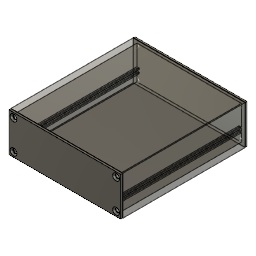
2230 Extruded aluminum box 94mm (Autodesk Fusion 360 design; units mm, degrees)
Autodesk Fusion 360 part; units mm, degrees
sketch "Sketch1" plane through (0, 0, 0) normal (0, 0, 1) x (1, 0, 0)
  line L0 (0, 0) -> (82.8, 0)
  line L1 (82.8, 0) -> (82.8, 28.8)
  line L2 (82.8, 28.8) -> (0, 28.8)
  line L3 (0, 28.8) -> (0, 0)
  line L4 (2.8, 2) -> (80, 2)
  line L5 (80, 26.8) -> (2.8, 26.8)
  line L6 (41.4, 28.8) -> (41.4, 0) construction
  line L7 (2.8, 9) -> (4.5, 9)
  line L8 (4.5, 9) -> (4.5, 8.1)
  line L9 (4.5, 8.1) -> (2.8, 8.1)
  line L10 (2.8, 8.1) -> (2.8, 9) construction
  line L11 (2.8, 11.7) -> (4.5, 11.7)
  line L12 (4.5, 11.7) -> (4.5, 10.8)
  line L13 (4.5, 10.8) -> (2.8, 10.8)
  line L14 (78.3, 8.1) -> (80, 8.1)
  line L15 (78.3, 9) -> (78.3, 8.1)
  line L16 (80, 9) -> (78.3, 9)
  line L17 (78.3, 10.8) -> (80, 10.8)
  line L18 (78.3, 11.7) -> (78.3, 10.8)
  line L19 (80, 11.7) -> (78.3, 11.7)
  line L20 (2.8, 26.8) -> (2.8, 11.7)
  line L21 (2.8, 8.1) -> (2.8, 2)
  line L22 (2.8, 10.8) -> (2.8, 9)
  line L23 (80, 11.7) -> (80, 26.8)
  line L24 (80, 2) -> (80, 8.1)
  line L25 (80, 9) -> (80, 10.8)
  dimension "d1" = 82.8
  dimension "d2" = 28.8
  dimension "d4" = 77.2
  dimension "d5" = 24.8
  dimension "d6" = 2
  dimension "d7" = 2.8
  dimension "d8" = 41.4
  dimension "d9" = 1.7
  dimension "d10" = 0.9
  dimension "d15" = 1.8
  dimension "d17" = 0.9
  dimension "d20" = 7
  measures "d4" distance of L0.start
  measures "d6" distance of L2 L5
  measures "d7" distance of L1 L24
  measures "d8" distance of L1 L6
  measures "d15" distance of L7 L13
  measures "d17" distance of L11 L13
  measures "d20" distance of L4 L7
extrude "Extrude1" add sketch "Sketch1" along normal blind 90.5 makes body 1
sketch "Sketch1 (2)" plane through (0, 0, 0) normal (0, 0, 1) x (1, 0, 0) in component "BackPanel"
  line L0 (0, 0) -> (82.8, 0)
  line L1 (82.8, 0) -> (82.8, 28.8)
  line L2 (82.8, 28.8) -> (0, 28.8)
  line L3 (0, 28.8) -> (0, 0)
  circle A0 centre (3.5, 3.5) radius 1.5
  circle A1 centre (79.3, 3.5) radius 1.5
  circle A2 centre (3.5, 25.3) radius 1.5
  circle A3 centre (79.3, 25.3) radius 1.5
  line L4 (0, 0) -> (3.5, 3.5) construction
  line L5 (0, 28.8) -> (3.5, 25.3) construction
  line L6 (82.8, 28.8) -> (79.3, 25.3) construction
  line L7 (82.8, 0) -> (79.3, 3.5) construction
  dimension "d1_1" = 82.8
  dimension "d2_1" = 28.8
  dimension "d3" = 3
  dimension "d8_1" = 75.8
  dimension "d9_1" = 21.9
  dimension "d29" = 3.5
  dimension "d30" = 3.5
  measures "d3" diameter of A0
  measures "d29" distance of L0.start
  measures "d30" distance of L0.start
extrude "Extrude1'" add sketch "Sketch1 (2)" along normal blind 1.5 separate body makes body 2 in component "BackPanel"
chamfer "Chamfer1" distance 1 angle 45 4 edges at (77.9015, 25.8424, 0) (77.9015, 4.0424, 0) (2.1015, 25.8424, 0) (2.1015, 4.0424, 0) on bodies 2 in component "BackPanel"
ref_plane "WorkPlane1" through (41.4, 14.4, 45.25) normal (0, 0, -1) x (-1, 0, 0)
mirror "MirrorComponent1" about plane through (0, 0, 0) normal (0, 0, 1) of bodies 2 makes body 3 in component "FrontPanel"
copy_body "CutPasteBodies1" bodies 1 removing the originals makes body 4 in component "Box"
component "Box" placed x (1, 0, 0) y (0, 1, 0) z (0, 0, 1) at (0, 0, 0)
component "BackPanel" placed x (1, 0, 0) y (0, 1, 0) z (0, 0, 1) at (0, 0, -1.5)
component "FrontPanel" placed x (1, 0, 0) y (0, 1, 0) z (0, 0, 1) at (0, 0, 92)
equation "d1 = BoxWidth"
equation "d2 = BoxHeight"
equation "d8 = d1 / 2"
equation "d17 = d10"
equation "d18 = BoxExtrusionDepth"
equation "d1_1 = BoxWidth"
equation "d2_1 = BoxHeight"
equation "d3 = ScrewShaftDiameter"
equation "BoxWidth = 82.8 mm"
equation "BoxHeight = 28.8 mm"
equation "BoxExtrusionDepth = TotalBoxDepth - ( PanelThickness * 2 )"
equation "ScrewShaftDiameter = 3 mm"
equation "ScrewHeadDiameter = 5 mm"
equation "TotalBoxDepth = 94 mm" comment "Including both panels"
equation "PanelThickness = 1.75 mm" comment "Drawing from adafruit.com says 1.5mm but mine are 2mm so I split the difference"
equation "ScrewInset = 3.5 mm" comment "Tolerance on this could be up to .05mm"
equation "d29 = ScrewInset"
equation "d30 = ScrewInset"
equation "d34 = ( ScrewHeadDiameter - ScrewShaftDiameter ) / 2"
